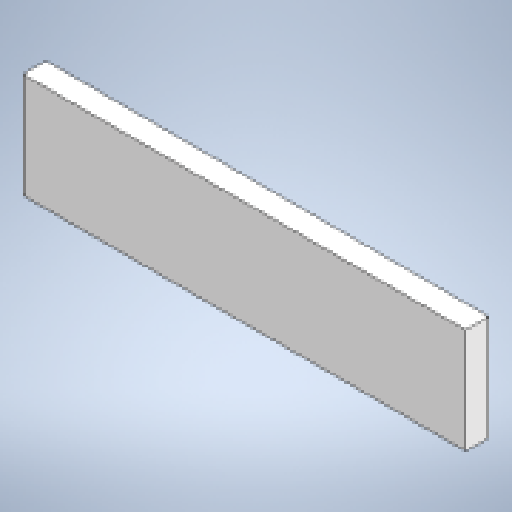
# Autodesk Inventor part: Back Plate
Saved by Autodesk Inventor 2023.2 (Build 272271000, 271)
## iProperties
Created: 2023-11-13
Part Number: Back Plate
Material: UHMW, White
Document SubType Name: Modeling
Designer: Nathan Cai
Density: 0.94 g/cm^3
Appearance: Smooth - White
Mass: 18.4124 g
Surface Area: 79.0321 cm^2
Volume: 19.5877 cm^3
Author: Nathan Cai
Autodesk Inventor part; units mm, degrees
ref_plane "YZ Plane" through (0, 0, 0) normal (1, 0, 0) x (0, 1, 0)
ref_plane "XZ Plane" through (0, 0, 0) normal (0, 1, 0) x (-1, 0, 0)
ref_plane "XY Plane" through (0, 0, 0) normal (0, 0, 1) x (1, 0, 0)
sketch "Sketch1" plane through (0, 0, 0) normal (0, 0, 1) x (1, 0, 0)
  line L0 (-60.325, -14.2875) -> (60.325, -14.2875)
  line L1 (60.325, -14.2875) -> (60.325, 14.2875)
  line L2 (60.325, 14.2875) -> (-60.325, 14.2875)
  line L3 (-60.325, 14.2875) -> (-60.325, -14.2875)
  line L4 (-60.325, -14.2875) -> (60.325, 14.2875) construction
  line L5 (60.325, -14.2875) -> (-60.325, 14.2875) construction
  point P0 (0, 0)
  dimension "d0" = 120.65
  dimension "d1" = 28.575
  constraints: 12 end point, 2 midpoint, 2 parallel, 1 horizontal, 1 perpendicular
  measures "d0" distance of L2.end L1.end
  measures "d1" distance of L1.end L0.end
extrude "Extrusion1" add sketch "Sketch1" along normal blind 6.35
body "Solid1"
